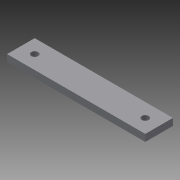
# Autodesk Inventor part: ArmPlate
Saved by Autodesk Inventor 2013 (Build 170138000, 138)
## iProperties
Created: 2014-01-22
Part Number: ArmPlate
Material: Generic
Document SubType Name: Modeling
Designer: 215152
Density: 1 g/cm^3
Author: 215152
Autodesk Inventor part; units mm, degrees
ref_plane "YZ Plane" through (0, 0, 0) normal (1, 0, 0) x (0, 1, 0)
ref_plane "XZ Plane" through (0, 0, 0) normal (0, 1, 0) x (-1, 0, 0)
ref_plane "XY Plane" through (0, 0, 0) normal (0, 0, 1) x (1, 0, 0)
sketch "Sketch1" plane through (0, 0, 0) normal (0, 1, 0) x (-1, 0, 0)
  line L0 (-63.5, -12.7) -> (63.5, -12.7)
  line L1 (63.5, -12.7) -> (63.5, 12.7)
  line L2 (63.5, 12.7) -> (-63.5, 12.7)
  line L3 (-63.5, 12.7) -> (-63.5, -12.7)
  line L4 (-63.5, -12.7) -> (63.5, 12.7) construction
  line L5 (63.5, -12.7) -> (-63.5, 12.7) construction
  point P0 (0, 0)
  dimension "d0" = 127
  dimension "d1" = 25.4
  constraints: 12 end point, 2 midpoint, 2 parallel, 1 horizontal, 1 perpendicular
  measures "d0" distance of L2.end L1.end
  measures "d1" distance of L1.end L0.end
extrude "Extrusion1" add sketch "Sketch1" along normal blind 6.35
sketch "Sketch2" plane through (0, 6.35, 0) normal (0, 1, 0) x (1, 0, 0)
  line L0 (-63.5, 12.7) -> (-63.5, -12.7) projected
  line L1 (63.5, -12.7) -> (63.5, 12.7) projected
  line L2 (-63.5, 0) -> (-50.8, 0)
  line L3 (-63.5, 0) -> (-50.8, 0) construction
  line L4 (63.5, 0) -> (50.8, 0)
  line L5 (63.5, 0) -> (76.2, 0) construction
  circle A0 centre (-50.8, 0) radius 3.175
  circle A1 centre (50.8, 0) radius 3.175
  point P0 (0, 0)
  dimension "d4" = 12.7
  dimension "d5" = 0
  dimension "d6" = 12.7
  dimension "d7" = 180
  dimension "d8" = 6.35
  dimension "d9" = 6.35
  constraints: 8 end point, 3 collinear, 2 centre point, 2 coincident, 2 horizontal, 2 midpoint, 1 perpendicular
  measures "d4" distance of L2.start L2.end
  measures "d5" distance between parallel lines of L2 L3
  measures "d6" distance of L4.start L4.end
  measures "d7" angle of L4 L5
  measures "d8" diameter of A0
  measures "d9" diameter of A1
extrude "Extrusion2" cut sketch "Sketch2" against normal blind 6.35
body "Solid1"
